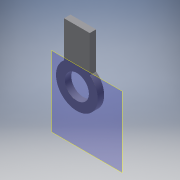
# Autodesk Inventor part: Part6
Saved by Autodesk Inventor 2016 (Build 200138000, 138)
## iProperties
Created: 2016-05-12
Part Number: Part6
Material: Generic
Document SubType Name: Modeling
Designer: ajar021
Density: 1 g/cm^3
Appearance: Default
Author: ajar021
Autodesk Inventor part; units mm, degrees
ref_plane "YZ Plane" through (0, 0, 0) normal (1, 0, 0) x (0, 1, 0)
ref_plane "XZ Plane" through (0, 0, 0) normal (0, 1, 0) x (-1, 0, 0)
ref_plane "Work Plane1" through (0, 0, -6.6) normal (0, 0, -1) x (-1, 0, 0)
sketch "Sketch1" plane through (0, 0, -6.6) normal (0, 0, -1) x (-1, 0, 0)
  circle A0 centre (3.0857, 5.1173) radius 10 projected
  line L0 (-6.9143, 5.1173) -> (-6.9143, 18.1173)
  line L1 (-6.9143, 18.1173) -> (13.0857, 18.1173)
  line L2 (13.0857, 18.1173) -> (13.0857, 5.1173)
  circle A1 centre (0, 0) radius 5
  point P0 (0, 0)
  dimension "d24" = 13
  dimension "d25" = 20
  constraints: 6 end point, 2 point on circle, 2 tangent, 1 centre point, 1 perpendicular, 1 vertical, 2 other
  measures "d24" distance of L0.start L0.end
  measures "d25" distance of L0.end L1.end
ref_plane "Work Plane2" through (-10, -10, -4.4) normal (0, 0, 1) x (1, 0, 0)
extrude "Extrusion1" add sketch "Sketch1" along normal blind 2 contours A0 A1 | A0 L0 L1 L2 | A0 A1 picked at (6.1055, 10.6249) picked at (0.8611, -2.5748)
sketch "Sketch9" plane through (0, 0, -8.6) normal (0, 0, -1) x (-1, 0, 0)
  circle A0 centre (3.0857, 5.1173) radius 5 construction
  arc A1 (-6.9143, 5.1173) -> (13.0857, 5.1173) centre (3.0857, 5.1173) ccw projected
  circle A2 centre (3.0857, 5.1173) radius 3.75
  dimension "d43" = 7.5
  constraints: 1 centre point, 1 coincident
  measures "d43" diameter of A2
extrude "Extrusion6" cut sketch "Sketch9" against normal up to surface (2 mm away)
sketch "Sketch10" plane through (0, 0, -8.6) normal (0, 0, -1) x (-1, 0, 0)
  arc A0 (-6.9143, 5.1173) -> (13.0857, 5.1173) centre (3.0857, 5.1173) ccw projected
  line L0 (3.0857, -4.8827) -> (3.0857, -2.8827)
  line L1 (3.0857, -2.8827) -> (4.5857, -2.8827)
  line L2 (4.5857, -2.8827) -> (3.0857, -2.8827)
  line L3 (-2.1325, -2.8827) -> (-2.1325, -5.7607)
  line L4 (4.5857, -2.8827) -> (4.5857, -3.3119)
  line L5 (-2.1325, -5.7607) -> (-2.1325, -7.2943)
  line L6 (4.5857, -3.3119) -> (4.5857, -2.7408)
  line L7 (-4, 15) -> (-4, 13) construction
  line L8 (4, 13) -> (4, 15) construction
  line L9 (13.0857, 18.1173) -> (-6.9143, 18.1173) projected
  line L10 (-6.9143, 18.1173) -> (13.0857, 18.1173)
  line L11 (-6.9143, 18.1173) -> (-6.9143, 5.1173)
  line L12 (13.0857, 18.1173) -> (13.0857, 5.1173)
  arc A1 (-6.9143, 5.1173) -> (13.0857, 5.1173) centre (3.0857, 5.1173) ccw
  circle A2 centre (3.0857, 5.1173) radius 6.5
  line L13 (3.0857, 5.1173) -> (3.0857, 11.6173) construction
  line L14 (3.0857, 11.6173) -> (7.0857, 11.6173)
  line L15 (7.0857, 11.6173) -> (3.0857, 11.6173)
  line L16 (3.0857, 11.6173) -> (-0.9143, 11.6173)
  line L17 (-0.9143, 10.2408) -> (-0.9143, 18.1173)
  line L18 (-0.9143, 18.1173) -> (7.0857, 18.1173)
  line L19 (7.0857, 18.1173) -> (7.0857, 10.2408)
  point P0 (5.6921, -0.9362)
  dimension "d31" = 2
  dimension "d37" = 1.5
  dimension "d44" = 4
  dimension "d45" = 4
  constraints: 34 end point, 7 point on circle, 6 point on line, 4 tangent, 3 perpendicular, 2 centre point, 2 collinear, 2 horizontal, 2 parallel, 2 vertical, 1 other
  measures "d31" distance of L0.start L0.end
  measures "d37" distance of L0.end L1.end
  measures "d44" distance of L13.end L14.end
  measures "d45" distance of L13.end L16.end
extrude "Extrusion8" cut sketch "Sketch10" against normal up to next contours A0 L11 L9 L17 A2 L19 L12
sketch "Sketch11" plane through (0, 0, -8.6) normal (0, 0, -1) x (-1, 0, 0)
  line L0 (7.0857, 18.1173) -> (-0.9143, 18.1173) projected
  line L1 (7.0857, 18.1173) -> (7.0857, 21.6173)
  line L2 (7.0857, 21.6173) -> (-0.9143, 21.6173)
  line L3 (-0.9143, 21.6173) -> (-0.9143, 18.1173)
  point P0 (0, 0)
  dimension "d46" = 3.5
  constraints: 6 end point, 2 perpendicular, 1 vertical
  measures "d46" distance of L0.start L1.end
extrude "Extrusion9" add sketch "Sketch11" against normal up to surface (2 mm away)
body "Solid1"
